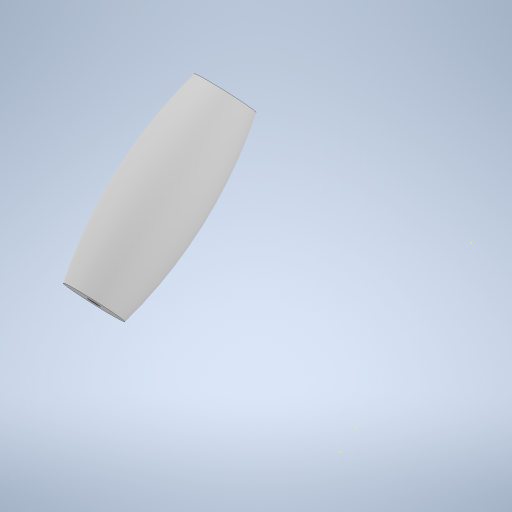
# Autodesk Inventor part: Part5
Saved by Autodesk Inventor 2024 (Build 280153000, 153)
## iProperties
Created: 2023-12-18
Part Number: Part5
Material: Generic
Document SubType Name: Modeling
Designer: SAHITYA
Density: 1 g/cm^3
Appearance: Default
Author: SAHITYA
Autodesk Inventor part; units mm, degrees
ref_plane "XZ Plane" through (0, 0, 0) normal (0, 1, 0) x (-1, 0, 0)
ref_plane "XY Plane" through (0, 0, 0) normal (0, 0, 1) x (1, 0, 0)
sketch "Sketch1" plane through (0, 0, 0) normal (0, 1, 0) x (-1, 0, 0)
  circle A0 centre (0, 0) radius 63.5
  dimension "d3" = 127
  constraints: 1 centre point
  measures "d3" diameter of A0
extrude "Extrusion1" add sketch "Sketch1" along normal blind 51
ref_plane "Work Plane1" through (-63.5, 0, 0) normal (1, 0, 0) x (0, 1, 0)
sketch "Sketch2" plane through (-63.5, 0, 0) normal (1, 0, 0) x (0, 1, 0)
  line L0 (51, -63.5) -> (51, 63.5)
  line L1 (51, -11.536887) -> (14.275563, -43.964498)
  line L2 (0, -63.5) -> (0, 63.5)
  line L3 (0, 7.464541) -> (44.188483, 46.482891)
  line L4 (51, -11.536887) -> (43.691421, -17.990349)
  line L5 (43.691421, -17.990349) -> (11.920531, 17.990349)
  line L6 (51, 0) -> (27.805976, 0)
  line L7 (51, -11.536887) -> (19.22911, 24.443811)
  line L8 (51, -11.536887) -> (43.691421, -17.990349)
  line L9 (43.691421, -17.990349) -> (36.382842, -24.443811)
  line L10 (36.382842, -24.443811) -> (4.611952, 11.536887)
  point P0 (0, 0)
  dimension "d6" = 48.5556
  dimension "d7" = 48.5556
  dimension "d8" = 9.75
  dimension "d9" = 48
  dimension "d10" = 9.75
  constraints: 18 end point, 7 point on line, 3 perpendicular, 2 midpoint, 1 collinear, 1 horizontal
  measures "d6" angle of L0 L1
  measures "d7" angle of L3 L2
  measures "d8" distance of L1.start L4.end
  measures "d9" distance of L4.end L5.end
  measures "d10" distance of L4.end L9.end
extrude "Extrusion2" cut sketch "Sketch2" along normal up to surface contours L1 L5 L6 L7 | L1 L10 L3 L5 | L6 L5 L3 L7 round surface about axis through (0, 0, 0) along (0, 1, 0) radius 63.5 far side no
sketch "Sketch3" plane through (0, 51, 0) normal (0, 1, 0) x (1, 0, 0)
  circle A0 centre (0, 0) radius 63.5
  constraints: 1 centre point, 1 coincident
extrude "Extrusion3" cut sketch "Sketch3" against normal through all
ref_plane "Work Plane2" through (-53.775, 0, 0) normal (1, 0, 0) x (0, 1, 0)
sketch "Sketch4" plane through (-53.775, 0, 0) normal (1, 0, 0) x (0, 1, 0)
  line L0 (36.382842, -24.443811) -> (51, -11.536887)
  line L1 (43.691421, -17.990349) -> (11.920531, 17.990349)
  line L2 (19.22911, 24.443811) -> (4.611952, 11.536887)
  line L3 (14.799002, 0) -> (36.382842, -24.443811)
  line L4 (25.590922, -12.221905) -> (40.20808, 0.685019)
  line L5 (40.81295, 0) -> (19.22911, 24.443811)
  line L6 (11.920531, 17.990349) -> (6.599886, 13.292228)
  line L7 (6.599886, 13.292228) -> (17.241177, 22.688469)
  line L8 (38.370775, -22.688469) -> (49.012066, -13.292228)
  line L9 (14.799002, 0) -> (40.81295, 0)
  arc A0 (49.012066, -13.292228) -> (17.241177, 22.688469) centre (-36.808713, -57.054652) ccw
  arc A1 (6.599886, 13.292228) -> (38.370775, -22.688469) centre (80.63629, 46.649071) ccw
  line L10 (14.799002, 0) -> (13.340961, 0)
  line L11 (13.340961, 0) -> (29.41616, 12.906924)
  line L12 (40.81295, 0) -> (25.590922, -12.221905)
  point P0 (0, 0)
  point P1 (13.87171, 0.426144)
  point P2 (21.805146, 6.795971)
  point P3 (33.201936, -6.110953)
  dimension "d16" = 7.098
  dimension "d17" = 14.196
  dimension "d18" = 14.196
  constraints: 16 end point, 6 point on circle, 6 point on line, 3 midpoint, 2 centre point, 2 coincident, 1 horizontal, 1 parallel, 1 perpendicular
  measures "d16" distance of L1.end L6.end
  measures "d17" distance of L6.end L7.end
  measures "d18" distance of L8.start L8.end
sketch "Sketch5" plane through (-63.5, 19.22911, 24.443811) normal (0, -0.6618935, 0.7495979) x (1, 0, 0)
  point P0 (63.5, -30.5933)
revolve "Revolution1" add sketch "Sketch4" angle 360 about axis through (-53.775, 43.691421, -17.990349) along (0, -0.6618935, 0.7495979) separate body contours L1 L12 A0 L0 | A1 L2 L1 L11
loft "Loft1" add bodies 2 section 1 edges at (-53.775, 26.195792, -12.906924) section 2 edges at (-53.775, 29.108087, 13.879837)
fillet "Face Fillet1" radius 2 1 edges at (-53.775, 26.1958, -12.9069)
sketch "Sketch6" plane through (-53.775, 43.691421, -17.990349) normal (0, 0.6618935, -0.7495979) x (-1, 0, 0)
  point P0 (-53.775, -20.8433)
sketch "Sketch7" plane through (0, 0, 0) normal (0, 1, 0) x (-1, 0, 0)
  point P0 (0, 0)
sketch "Sketch8" plane through (-53.775, 11.920531, 17.990349) normal (0, -0.6618935, 0.7495979) x (1, 0, 0)
  circle A0 centre (0, 0) radius 7.098
  line L0 (0, 7.098) -> (0, -16.474926)
  line L1 (0, -16.474926) -> (25.907783, -18.985487)
  line L2 (25.907783, -18.985487) -> (15.564277, 30.623181)
  line L3 (15.564277, 30.623181) -> (0, 22.890656)
  line L4 (0, 22.890656) -> (0, 7.098)
  point P0 (53.775, -20.8433)
  constraints: 10 end point, 1 collinear, 1 point on line, 1 vertical, 1 vertical alignment, 1 other
extrude "Extrusion4" cut sketch "Sketch8" against normal through all contours A0 L0 | A0 L4 L3 L2 L1 L0 picked at (1.475177, 1.849813) bodies 2
sketch "Sketch9" plane through (-53.775, 6.599886, 13.292228) normal (1, 0, 0) x (0, 0.6618935, -0.7495979)
  line L0 (0, 14.196) -> (0, 0)
  line L1 (0, 7.098) -> (48, 7.098)
  line L2 (48, 14.196) -> (48, 0)
  arc A0 (48, 14.196) -> (32.676778, 16.841915) centre (24, -79.101138) ccw
  line L3 (48, 7.098) -> (48, 14.196)
  line L4 (0, 7.098) -> (0, 14.196)
  arc A1 (48, 14.196) -> (0, 14.196) centre (24, -85.055258) ccw
  line L5 (0, 14.196) -> (0, 20.824177)
  line L6 (0, 20.824177) -> (48, 20.824177)
  line L7 (48, 20.824177) -> (48, 14.196)
  point P0 (5.595404, -13.7453)
  constraints: 12 end point, 2 midpoint, 2 perpendicular, 2 point on circle, 2 vertical, 1 centre point, 1 collinear
revolve "Revolution2" cut sketch "Sketch9" angle 360 about axis through (-53.775, 11.920531, 17.990349) along (0, 0.6618935, -0.7495979) bodies 2 contours L5 L6 L7 A1
sketch "Sketch10" plane through (-53.775, 6.599886, 13.292228) normal (1, 0, 0) x (0, 0.6618935, -0.7495979)
  line L0 (48, 14.196) -> (48, 0)
  line L1 (48, 7.098) -> (0, 7.098)
  line L2 (0, 0) -> (0, 14.196)
  line L3 (0, 0) -> (0, 7.098)
  line L4 (48, 7.098) -> (48, 0)
  line L5 (48, 0) -> (48, -9.635667)
  line L6 (48, -9.635667) -> (0, -9.635667)
  line L7 (0, -9.635667) -> (0, 0)
  arc A0 (0, 0) -> (23.49985, -2.85928) centre (24, 99.251258) ccw
  arc A1 (29.144199, -2.730845) -> (48, 0) centre (24, 99.251258) ccw
  arc A2 (0, 0) -> (48, 0) centre (24, 99.251258) ccw
  point P0 (5.595404, -13.7453)
  point P1 (23.49985, -2.85928)
  constraints: 12 end point, 2 midpoint, 2 perpendicular, 2 point on circle, 2 point on line, 1 centre point, 1 collinear, 1 vertical
revolve "Revolution3" add sketch "Sketch10" angle 360 about axis through (-53.775, 43.691421, -17.990349) along (0, -0.6618935, 0.7495979) bodies 2 contours L0 A1 A2 A0 L2 L1
revolve "Revolution4" cut sketch "Sketch10" angle 360 about axis through (-53.775, 43.691421, -17.990349) along (0, -0.6618935, 0.7495979) bodies 2 contours L5 L6 L7 A0 A2 A1
sketch "Sketch11" plane through (-53.775, 11.920531, 17.990349) normal (0, -0.6618935, 0.7495979) x (1, 0, 0)
  circle A0 centre (0, 0) radius 7.098 projected
  circle A1 centre (0, 0) radius 1.5
  point P0 (53.775, -20.8433)
  dimension "d30" = 3
  constraints: 1 centre point, 1 coincident
  measures "d30" diameter of A1
extrude "Extrusion5" cut sketch "Sketch11" against normal through all contours A1 bodies 2
body "Solid1"
body "Solid3"
